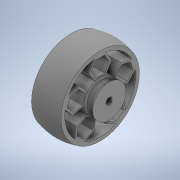
# Autodesk Inventor part: PulleyedWheelV1
Saved by Autodesk Inventor 2020 (Build 240168000, 168)
## iProperties
Created: 2023-12-21
Part Number: PulleyedWheelV1
Material: H TPU
Document SubType Name: Modeling
Designer: smz3rm
Density: 0.941117 g/cm^3
Appearance: Generic(1)
Mass: 7.7724 g
Surface Area: 68.3098 cm^2
Volume: 8.2587 cm^3
d0: 3.000 mm
d1: 1.000 mm
d3: 34.500 mm
d4: 3.000 mm
d6: 14.600 mm
d7: 4.000 mm
d8: 0.00 deg
d9: 34.500 mm
d10: 1.600 mm
d11: 0.800 mm
d16: 13.000 mm
d17: 0.00 deg
d20: 2.000 mm
d24: 1.000 mm
d26: 45.00 deg
Roundedness: 1.000 mm
BaseThickness: 3.000 mm
TopThickness: 1.778 mm
SideThickness: 4.000 mm
BodyWidth: 130.000 mm
BodyLength: 150.000 mm
BodyHeight: 35.000 mm
DriveMotorHeight: 17.500 mm
WheelDia: 36.500 mm
WheelWidth: 13.000 mm
WheelGrooveWidth: 4.000 mm
WheelGrooveDia: 14.600 mm
WheelSlotWidth: 20.000 mm
WheelPulleyDia: 2.000 mm
WheeGuardlSlotWidth: 20.000 mm
Author: smz3rm
Autodesk Inventor part; units mm, degrees
ref_plane "YZ Plane" through (0, 0, 0) normal (1, 0, 0) x (0, 1, 0)
ref_plane "XZ Plane" through (0, 0, 0) normal (0, 1, 0) x (-1, 0, 0)
ref_plane "XY Plane" through (0, 0, 0) normal (0, 0, 1) x (1, 0, 0)
sketch "Sketch1" plane through (0, 0, 0) normal (1, 0, 0) x (0, 1, 0)
  circle A0 centre (0, 0) radius 1.5
  line L0 (-24.15, 0) -> (24.15, 0) projected
  line L1 (1.118, -1) -> (-1.118, -1)
  circle A1 centre (0, 0) radius 7.3
  circle A2 centre (0, 0) radius 17.25
  circle A3 centre (0, 0) radius 14.25
  dimension "d0" = 3
  dimension "d1" = 1
  dimension "d3" = 34.5
  dimension "d4" = 3
  dimension "d6" = 14.6
  constraints: 4 centre point, 4 coincident, 2 end point, 2 point on circle, 1 horizontal
  measures "d0" diameter of A0
  measures "d1" distance between parallel lines of L0 L1
  measures "d3" diameter of A2
  measures "d4" radial gap between concentric circles of A2 A3
  measures "d6" diameter of A1
extrude "Extrusion1" add sketch "Sketch1" along normal blind 4 contours L1 A0 | A0 L0 A1 | L0 A1 A0
sketch "Sketch3" plane through (0, 0, 0) normal (0, 0, 1) x (1, 0, 0)
  line L0 (0, 7.3) -> (4, 7.3) projected
  line L1 (-0.8, 0) -> (4.8, 0) projected
  circle A0 centre (1.3858, 6.3) radius 1
  line L2 (0.4001, 6.1312) -> (0.2, 7.3)
  line L3 (0, 7.3) -> (4, 7.3) projected
  line L4 (0, 10) -> (4, 10) projected
  line L5 (0, 7.3) -> (4, 7.3) projected
  line L6 (3.8, 7.3) -> (2.0929, 5.5929)
  line L7 (3.8, 7.3) -> (3.8, 7.3)
  line L8 (3.8, 7.3) -> (4, 7.3)
  line L9 (4, -7.3) -> (4, 7.3) projected
  line L10 (4, 7.3) -> (4, 7.3)
  line L11 (0, -7.3) -> (0, 7.3) projected
  line L12 (0.2, 7.3) -> (0, 7.3)
  point P0 (0, 0)
  point P1 (1.3858, 7.3)
  point P2 (3.8, 7.3)
  dimension "d20" = 2
  dimension "d26" = 45
  dimension "d28" = 0.2
  constraints: 12 end point, 3 perpendicular, 3 tangent, 2 collinear, 2 point on circle, 2 point on line, 1 centre point, 1 vertical, 3 other
  measures "d20" diameter of A0
  measures "d26" angle of L0 L6
  measures "d28" distance of L0.end L6.start
revolve "Revolution1" cut sketch "Sketch3" angle 360 about axis through (-10, 0, 0) along (-1, 0, 0) contours L0 A0 L2 | L0 L6 A0 | A0
sketch "Sketch2" plane through (0, 0, 0) normal (-1, 0, 0) x (0, 0, 1)
  circle A0 centre (0, 0) radius 17.25
  circle A1 centre (0, 0) radius 15.65
  circle A2 centre (0, 0) radius 7.3 projected
  line L0 (-1, 1.118) -> (-1, -1.118) projected
  arc A3 (-1, -1.118) -> (-1, 1.118) centre (0, 0) ccw projected
  line L1 (2.4786, 15.4525) -> (4.9572, 11.1594)
  line L2 (4.9572, 11.1594) -> (2.4786, 6.8663)
  line L3 (2.4786, 6.8663) -> (-2.4786, 6.8663)
  line L4 (-2.4786, 6.8663) -> (-4.9572, 11.1594)
  line L5 (-4.9572, 11.1594) -> (-2.4786, 15.4525)
  line L6 (-2.4786, 15.4525) -> (2.4786, 15.4525)
  line L7 (0, -24.15) -> (0, 24.15) projected
  line L8 (-2.0167, 14.6525) -> (-4.0335, 11.1594)
  line L9 (-4.0335, 11.1594) -> (-2.0167, 7.6663)
  line L10 (-2.0167, 7.6663) -> (2.0167, 7.6663)
  line L11 (2.0167, 7.6663) -> (4.0335, 11.1594)
  line L12 (4.0335, 11.1594) -> (2.0167, 14.6525)
  line L13 (2.0167, 14.6525) -> (-2.0167, 14.6525)
  line L14 (-13.9302, 7.1324) -> (-9.0814, 8.163)
  line L15 (-15.4621, 2.4178) -> (-13.9302, 7.1324)
  line L16 (-12.1451, -1.2661) -> (-15.4621, 2.4178)
  line L17 (-7.2962, -0.2355) -> (-12.1451, -1.2661)
  line L18 (-11.8596, -0.3876) -> (-7.9143, 0.451)
  line L19 (-7.9143, 0.451) -> (-6.6679, 4.287)
  line L20 (-6.6679, 4.287) -> (-9.3668, 7.2845)
  line L21 (-9.0814, 8.163) -> (-5.7643, 4.4791)
  line L22 (-5.7643, 4.4791) -> (-7.2962, -0.2355)
  line L23 (-9.3668, 7.2845) -> (-13.3121, 6.4459)
  line L24 (-13.3121, 6.4459) -> (-14.5585, 2.6098)
  line L25 (-14.5585, 2.6098) -> (-11.8596, -0.3876)
  line L26 (-11.088, -11.0444) -> (-10.5698, -6.1144)
  line L27 (-7.0775, -13.9582) -> (-11.088, -11.0444)
  line L28 (-2.5489, -11.9419) -> (-7.0775, -13.9582)
  line L29 (-2.0307, -7.0119) -> (-2.5489, -11.9419)
  line L30 (-3.2962, -11.399) -> (-2.8746, -7.3876)
  line L31 (-2.8746, -7.3876) -> (-6.1377, -5.0168)
  line L32 (-6.1377, -5.0168) -> (-9.8225, -6.6573)
  line L33 (-10.5698, -6.1144) -> (-6.0412, -4.0981)
  line L34 (-6.0412, -4.0981) -> (-2.0307, -7.0119)
  line L35 (-9.8225, -6.6573) -> (-10.2441, -10.6687)
  line L36 (-10.2441, -10.6687) -> (-6.9809, -13.0395)
  line L37 (-6.9809, -13.0395) -> (-3.2962, -11.399)
  line L38 (7.0775, -13.9582) -> (2.5489, -11.9419)
  line L39 (11.088, -11.0444) -> (7.0775, -13.9582)
  line L40 (10.5698, -6.1144) -> (11.088, -11.0444)
  line L41 (6.0412, -4.0981) -> (10.5698, -6.1144)
  line L42 (9.8225, -6.6573) -> (6.1377, -5.0168)
  line L43 (6.1377, -5.0168) -> (2.8746, -7.3876)
  line L44 (2.8746, -7.3876) -> (3.2962, -11.399)
  line L45 (2.5489, -11.9419) -> (2.0307, -7.0119)
  line L46 (2.0307, -7.0119) -> (6.0412, -4.0981)
  line L47 (3.2962, -11.399) -> (6.9809, -13.0395)
  line L48 (6.9809, -13.0395) -> (10.2441, -10.6687)
  line L49 (10.2441, -10.6687) -> (9.8225, -6.6573)
  line L50 (15.4621, 2.4178) -> (12.1451, -1.2661)
  line L51 (13.9302, 7.1324) -> (15.4621, 2.4178)
  line L52 (9.0814, 8.163) -> (13.9302, 7.1324)
  line L53 (5.7643, 4.4791) -> (9.0814, 8.163)
  line L54 (9.3668, 7.2845) -> (6.6679, 4.287)
  line L55 (6.6679, 4.287) -> (7.9143, 0.451)
  line L56 (7.9143, 0.451) -> (11.8596, -0.3876)
  line L57 (12.1451, -1.2661) -> (7.2962, -0.2355)
  line L58 (7.2962, -0.2355) -> (5.7643, 4.4791)
  line L59 (11.8596, -0.3876) -> (14.5585, 2.6098)
  line L60 (14.5585, 2.6098) -> (13.3121, 6.4459)
  line L61 (13.3121, 6.4459) -> (9.3668, 7.2845)
  point P0 (0, 11.1594)
  point P1 (2.4786, 6.8663)
  dimension "d9" = 34.5
  dimension "d10" = 1.6
  dimension "d11" = 0.8
  dimension "d31" = 360
  constraints: 120 end point, 2 centre point, 2 coincident, 2 point on circle, 1 point on line, 141 other
  measures "d9" diameter of A0
  measures "d10" radial gap between concentric circles of A0 A1
  measures "d11" distance between parallel lines of L5 L8
extrude "Extrusion2" add sketch "Sketch2" along normal blind 13 contours A0 L7 A1 | L7 A1 A0 | L7 L6 A1 | A1 L6 L7 | L1 L2 A2 L7 L10 L11 L12 L13 L6 | L6 L7 L13 L8 L9 L10 A2 L4 L5 | A1 L27 | L27 L26 L33 A2 L29 L28 | L39 A1 | L38 L45 A2 L41 L40 L39 | L7 A3 L3 A2 L58 L46 | A2 L34 L22 L3 L7 A3 L0 | A1 L51 | L51 L50 L57 A2 L53 L52 | L15 A1 | L14 L21 A2 L17 L16 L15 | A2 L34 | L46 A2 | L7 A3 | A3 L0 L7 | L3 L7 A2 | A2 L7 L3 | A2 L58 | L22 A2
sketch "Sketch4" plane through (0, 0, 0) normal (0, 0, 1) x (1, 0, 0)
  line L0 (0, 17.25) -> (-13, 17.25) projected
  line L1 (-13, 17.25) -> (-13, -17.25) projected
  arc A0 (0, 17.25) -> (-13, 17.25) centre (-6.5, -3.375) ccw
  line L2 (-15.6, 0) -> (2.6, 0) projected
  point P0 (0, 0)
  point P1 (-6.5, 18.25)
  dimension "d24" = 1
  constraints: 3 point on circle, 1 centre point
  measures "d24" distance from line of L0 point (-6.5, 18.25)
revolve "Revolution2" add sketch "Sketch4" angle 360 about axis through (-10, 0, 0) along (1, 0, 0)
equation "\"d6\" = WheelGrooveDia"
equation "\"d7\" = WheelGrooveWidth"
equation "\"d20\" = WheelPulleyDia"
equation "\"d9\" = WheelDia - 2 * Roundedness"
equation "\"d16\" = WheelWidth"
equation "\"d24\" = Roundedness"
equation "\"Roundedness\" = 1"
equation "\"WheelGrooveDia\" = 14.6"
equation "\"WheelGrooveWidth\" = 4"
equation "\"WheelPulleyDia\" = 2"
equation "\"WheelDia\" = 36.5"
equation "\"WheelWidth\" = 13"
body "Solid1"
